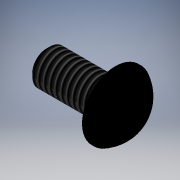
# Autodesk Inventor part: 3042
Saved by Autodesk Inventor 2017.3 (Build 213256000, 256)
## iProperties
Part Number: 3042
Material: Generic
Catalog Web Link: www.cadenas.de
Description: 3005, 3024, 3032, 3042, 3050, 3051, 3054, 3059, 3061, 3063, 3065, 3104, 3111, 3114, 3117, 3118-Button Head Socket Cap Screws
Vendor: 8020
Document SubType Name: Modeling
Designer: partserver
Manufacturer: 8020
Mass: 0.275004 g
Surface Area: 3.30369 cm^2
Volume: 0.275004 cm^3
Density: 1 g/cm^3
Appearance: PSOLRGB-0-0-0
Category: PARTsolutions
Company: 8020
Title: 3042
Author: Cadenas PARTsolutions
Comments: Button Head Socket Cap Screws
PSOL_IDENT_0: {$CADENAS_DATA\23d-libs\8020\inch\fastening_options\3005.prj},238 {VTYP=3D},{NB=3042},{LINA=3042},{N
PSOL_IDENT_1: N=3005, 3024, 3032, 3042, 3050, 3051, 3054, 3059, 3061, 3063, 3065, 3104, 3111, 3114, 3117, 3118},{D
PSOL_IDENT_2: ATE=20.05.2021 05:17:54},{GEOMDATE=03.08.2012 12:04:00},{VERSION=},{LINEID=60},{WBVAR=L},{WBNUMERIC=
PSOL_IDENT_3: L}  {NB=3042},{LINA=3042},{KT=DUMMY},{PN=3042},{FIN=Black Zinc},{THRD=10-32},{THRD1=0.1900},{L=0.375
PSOL_IDENT_4: 00000},{L1=[0.375,0.5,0.625,0.75]},{TT=UNF},{A=0.361},{A1=0.3610},{H=0.101},{H1=0.013},{J=0.125},{J1=
PSOL_IDENT_5: 0.12500},{T=0.0883},{R=0.201},{W=.004}
NB: 3042
NN: 3005, 3024, 3032, 3042, 3050, 3051, 3054, 3059, 3061, 3063, 3065, 3104, 3111, 3114, 3117, 3118
NT: Button Head Socket Cap Screws
NBSYN: $PN.
LINA: 3042
CATALOG: 80/20
PN: 3042
FIN: Black Zinc
THRD: 10-32
L: 0
A: 0.361
H: 0.101
J: 0.125
W: .004
SUPPLIER: 8020
ARTICLENO: 3042
BOMINFO: 3042
CREATOR: CADENAS GmbH
Autodesk Inventor part; units mm, degrees
sketch "Sketch_2" plane through (0, 0, 0) normal (0, 0, 1) x (1, 0, 0)
  line L0 (9.525, 0) -> (-2.5654, 0)
  line L1 (-2.5654, 0) -> (-2.5654, 2.413)
  arc A0 (-0.3302, 4.5847) -> (-2.5654, 2.413) centre (1.9401, 0.0119) ccw
  line L2 (-0.3302, 4.5847) -> (0, 4.5847)
  line L3 (0, 4.5847) -> (0, 2.413)
  line L4 (0, 2.413) -> (9.0526, 2.413)
  line L5 (9.0526, 2.413) -> (9.525, 1.9406)
  line L6 (9.525, 1.9406) -> (9.525, 0)
  line L7 (9.525, 0) -> (-2.5654, 0)
  constraints: 16 end point, 2 point on circle, 1 centre point
revolve "Revolution1" add sketch "Sketch_2" angle 360 about axis through (9.525, 0, 0) along (1, 0, 0)
thread "Thread1" size "10-32 UNF" class "2A" standard "ANSI Unified Screw Threads" length 8.2343
sketch "Sketch_3" plane through (-2.5654, 0, 0) normal (1, 0, 0) x (0, 0, -1)
  line L0 (-1.8331, 0) -> (-0.9165, -1.5875)
  line L1 (-0.9165, -1.5875) -> (0.9165, -1.5875)
  line L2 (0.9165, -1.5875) -> (1.8331, 0)
  line L3 (1.8331, 0) -> (0.9165, 1.5875)
  line L4 (0.9165, 1.5875) -> (-0.9165, 1.5875)
  line L5 (-0.9165, 1.5875) -> (-1.8331, 0)
  constraints: 12 end point
extrude "Extrusion1" cut sketch "Sketch_3" along normal mid plane 4.4856
ref_plane "screw_XY" through (0, 0, 0) normal (1, 0, 0) x (0, 0, -1)
ref_plane "screw_YZ" through (0, 0, 0) normal (0, 0, -1) x (0, 1, 0)
ref_plane "screw_ZX" through (0, 0, 0) normal (0, 1, 0) x (1, 0, 0)
ref_plane "to_nut_XY" through (9.525, 0, 0) normal (1, 0, 0) x (0, 0, -1)
ref_plane "to_nut_YZ" through (9.525, 0, 0) normal (0, 0, -1) x (0, 1, 0)
ref_plane "to_nut_ZX" through (9.525, 0, 0) normal (0, 1, 0) x (1, 0, 0)
body "Solid1"
